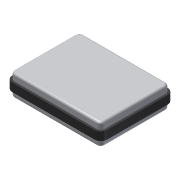
# Autodesk Inventor part: D-Link Wireless Bridge Radio
Saved by Autodesk Inventor 2013 (Build 170138000, 138)
## iProperties
Created: 2013-12-22
Part Number: D-Link Wireless Bridge Radio
Material: Generic
Document SubType Name: Modeling
Designer: Nemo
Mass: 226.796 g
Surface Area: 590.038 cm^2
Volume: 498.265 cm^3
Density: 0.455171 g/cm^3
Author: Nemo
Autodesk Inventor part; units mm, degrees
ref_plane "YZ Plane" through (0, 0, 0) normal (1, 0, 0) x (0, 1, 0)
ref_plane "XZ Plane" through (0, 0, 0) normal (0, 1, 0) x (-1, 0, 0)
ref_plane "XY Plane" through (0, 0, 0) normal (0, 0, 1) x (1, 0, 0)
sketch "Sketch2" plane through (0, 0, 0) normal (0, 1, 0) x (-1, 0, 0)
  line L0 (-69.215, 52.705) -> (69.215, 52.705)
  line L1 (69.215, 52.705) -> (69.215, -52.705)
  line L2 (69.215, -52.705) -> (-69.215, -52.705)
  line L3 (-69.215, -52.705) -> (-69.215, 52.705)
  point P0 (0, 0)
  point P1 (-69.215, 0)
  point P2 (0, -52.705)
  dimension "d0" = 138.43
  dimension "d1" = 105.41
  constraints: 8 end point, 2 midpoint, 2 parallel, 1 horizontal, 1 horizontal alignment, 1 perpendicular, 1 vertical alignment
  measures "d0" distance of L1.end L2.end
  measures "d1" distance of L0.end L1.end
extrude "Extrusion1" add sketch "Sketch2" along normal mid plane 33.02
fillet "Fillet1" radius 6.35 4 edges at (69.215, 0, 52.705) (69.215, 0, -52.705) (-69.215, 0, -52.705) (-69.215, 0, 52.705)
fillet "Fillet2" radius 3.175 16 edges at (0, -16.51, 52.705) (0, 16.51, 52.705) (-67.3551, -16.51, 50.8451) (-69.215, -16.51, 0) (-67.3551, -16.51, -50.8451) (0, -16.51, -52.705) (67.3551, -16.51, -50.8451) (69.215, -16.51, 0) (67.3551, -16.51, 50.8451) (67.3551, 16.51, 50.8451) (69.215, 16.51, 0) (67.3551, 16.51, -50.8451) (0, 16.51, -52.705) (-67.3551, 16.51, -50.8451) (-69.215, 16.51, 0) (-67.3551, 16.51, 50.8451)
sketch "Sketch3" plane through (0, 0, 0) normal (0, 1, 0) x (-1, 0, 0)
  arc A0 (62.865, -52.705) -> (69.215, -46.355) centre (62.865, -46.355) ccw projected
  line L0 (62.865, -52.705) -> (-62.865, -52.705) projected
  arc A1 (-69.215, -46.355) -> (-62.865, -52.705) centre (-62.865, -46.355) ccw projected
  line L1 (-69.215, -46.355) -> (-69.215, 46.355) projected
  arc A2 (-62.865, 52.705) -> (-69.215, 46.355) centre (-62.865, 46.355) ccw projected
  line L2 (-62.865, 52.705) -> (62.865, 52.705) projected
  arc A3 (69.215, 46.355) -> (62.865, 52.705) centre (62.865, 46.355) ccw projected
  line L3 (69.215, 46.355) -> (69.215, -46.355) projected
  line L4 (62.865, 55.88) -> (-62.865, 55.88)
  arc A4 (-62.865, 55.88) -> (-72.39, 46.355) centre (-62.865, 46.355) ccw
  line L5 (-72.39, 46.355) -> (-72.39, -46.355)
  arc A5 (-72.39, -46.355) -> (-62.865, -55.88) centre (-62.865, -46.355) ccw
  line L6 (-62.865, -55.88) -> (62.865, -55.88)
  arc A6 (62.865, -55.88) -> (72.39, -46.355) centre (62.865, -46.355) ccw
  line L7 (72.39, -46.355) -> (72.39, 46.355)
  arc A7 (72.39, 46.355) -> (62.865, 55.88) centre (62.865, 46.355) ccw
  point P0 (0, 0)
  dimension "d6" = 3.175
  constraints: 8 end point, 8 point on circle, 4 centre point, 7 other
  measures "d6" distance between parallel lines of L4 L2
extrude "Extrusion2" add sketch "Sketch3" along normal mid plane 12.7 separate body
body "Solid1"
body "Solid2"
